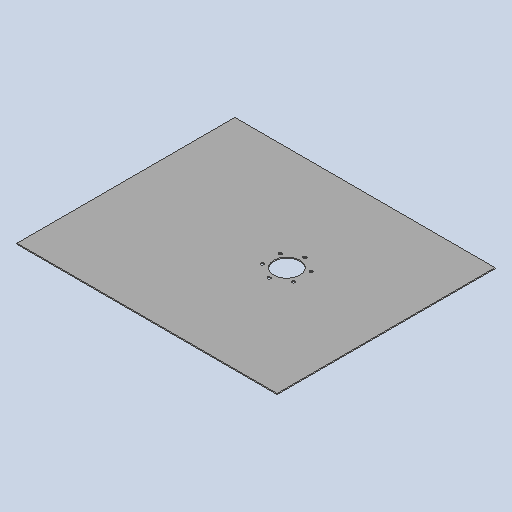
# Autodesk Inventor part: TRM 015 left board main
Saved by Autodesk Inventor 2025 (Build 290162010, 162A)
## iProperties
Created: 2024-08-07
Part Number: TRM 015 left board main
Material: AISI 304
Document SubType Name: Sheet Metal
Designer: pokla
Density: 8.02768 g/cm^3
Flat Pattern Width: 80 cm
Flat Pattern Length: 67 cm
Flat Pattern Area: 5360 cm^2
Sheet Metal Rule: AISI304 2mm Die16
Sheet Metal Width: 800.000 mm
Sheet Metal Length: 670.000 mm
Sheet Metal Area: 536000.000 mm^2
Appearance: Default
Stock Number: ТРМ 015 левый борт основное
Mass: 12776.1 g
Surface Area: 10711.4 cm^2
Volume: 1591.51 cm^3
Author: pokla
Autodesk Inventor part; units mm, degrees
ref_plane "YZ Plane" through (0, 0, 0) normal (1, 0, 0) x (0, 1, 0)
ref_plane "XZ Plane" through (0, 0, 0) normal (0, 1, 0) x (-1, 0, 0)
ref_plane "XY Plane" through (0, 0, 0) normal (0, 0, 1) x (1, 0, 0)
sketch "Sketch1" plane through (0, 0, 0) normal (0, 0, 1) x (1, 0, 0)
  line L0 (320, 0) -> (320, 670)
  line L1 (320, 670) -> (-480, 670)
  line L2 (-480, 670) -> (-480, 0)
  circle A0 centre (0, 350) radius 40
  line L3 (320, 0) -> (-480, 0)
  point P0 (0, 0)
  dimension "d14" = 80
  dimension "d15" = 320
  dimension "d17" = 320
  dimension "d26" = 800
  dimension "d27" = 670
  measures "d14" diameter of A0
  measures "d15" distance from line of A0.centre L1
  measures "d17" distance from line of L0 A0.centre
  measures "d26" distance between parallel lines of L2 L0
  measures "d27" distance between parallel lines of L3 L1
extrude "Plate1" add sketch "Sketch1" along normal blind 3
sketch "Sketch2" plane through (0, 0, 0) normal (0, 0, -1) x (-1, 0, 0)
  line L0 (-300, 650) -> (-100, 650) construction
  line L1 (-100, 650) -> (-100, 630) construction
  line L2 (-100, 630) -> (-300, 630) construction
  line L3 (-300, 630) -> (-300, 650) construction
  line L4 (-320, 670) -> (480, 670) projected
  line L5 (-320, 0) -> (-320, 670) projected
  point P0 (0, 0)
  point P1 (-48, 100)
  point P2 (480, 670)
  point P3 (-251, -525)
  point P4 (-50, 98)
  point P5 (-320, 0)
  dimension "d6" = 200
  dimension "d9" = 20
  dimension "d10" = 20
  dimension "d11" = 20
  constraints: 4 other
  measures "d6" distance of L0.start L0.end
  measures "d9" distance of L0.end L1.end
  measures "d11" length of L3
mark "Mark1"
sketch "Sketch3" plane through (0, 0, 3) normal (0, 0, 1) x (1, 0, 0)
  circle A0 centre (0, 405) radius 5
  circle A1 centre (0, 350) radius 40 projected
  point P0 (0, 0)
  dimension "d19" = 10
  dimension "d20" = 55
  constraints: 1 centre point, 1 vertical alignment
  measures "d19" diameter of A0
  measures "d20" distance of A1.centre A0.centre
extrude "Cut1" cut sketch "Sketch3" against normal through all contours A0
pattern_circular "Circular Pattern1" count 6 over 360 about axis through (0, 350, 0) along (0, 0, 1) of "Cut1"
equation "\"d2\" = Thickness"
equation "\"BendReliefWidth\" = Thickness"
equation "\"BendReliefDepth\" = 0.5 * Thickness"
equation "\"CornerReliefSize\" = 4 * Thickness"
equation "\"MinimumRemnant\" = 2 * Thickness"
equation "\"TransitionRadius\" = BendRadius"
equation "\"JacobiRadiusSize\" = BendRadius"
equation "\"GapSize\" = Thickness"
equation "\"Thickness\" = 3"
equation "\"BendRadius\" = 2.75"
body "Solid1"
